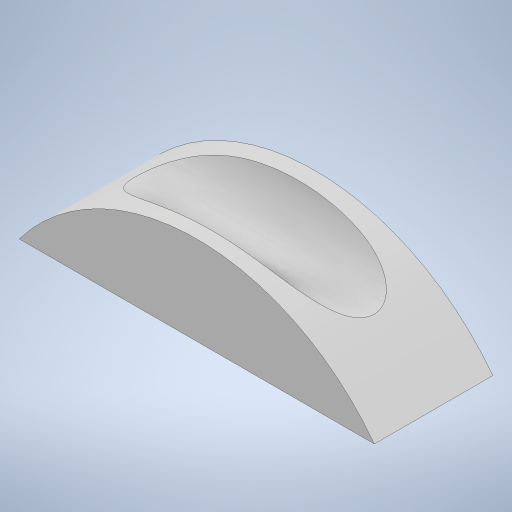
# Autodesk Inventor part: cuff
Saved by Autodesk Inventor 2024 (Build 280153000, 153)
## iProperties
Created: 2023-09-09
Part Number: cuff
Material: Generic
Document SubType Name: Modeling
Designer: Pintu
Density: 1 g/cm^3
Appearance: Default
Author: Pintu
Autodesk Inventor part; units mm, degrees
ref_plane "YZ Plane" through (0, 0, 0) normal (1, 0, 0) x (0, 1, 0)
ref_plane "XZ Plane" through (0, 0, 0) normal (0, 1, 0) x (-1, 0, 0)
ref_plane "XY Plane" through (0, 0, 0) normal (0, 0, 1) x (1, 0, 0)
sketch "Sketch1" plane through (0, 0, 0) normal (0, 0, 1) x (1, 0, 0)
  arc A0 (120, 0) -> (-120, 0) centre (0, -90) ccw
  line L0 (-120, 0) -> (120, 0)
  point P0 (0, 0)
  dimension "d0" = 240
  dimension "d1" = 150
  dimension "d2" = 120
  constraints: 2 end point, 2 horizontal alignment, 2 point on circle, 1 centre point, 1 horizontal
  measures "d0" distance of L0.start L0.end
  measures "d1" radius of A0
  measures "d2" distance of L0.start point (0, 0)
extrude "Extrusion1" add sketch "Sketch1" along normal mid plane 80
sketch "Sketch2" plane through (0, 0, 0) normal (1, 0, 0) x (0, 1, 0)
  line L0 (60, -40) -> (60, 40) projected
  arc A0 (60, 30) -> (60, -28.5626) centre (66.5274, 0.7187) ccw
  point P0 (0, 0)
  point P1 (60, 0)
  dimension "d5" = 30
  dimension "d6" = 30
  constraints: 2 point on circle, 2 point on line, 1 centre point, 1 midpoint
  measures "d5" radius of A0
  measures "d6" distance of point (60, 0) A0.start
extrude "Extrusion2" cut sketch "Sketch2" along normal mid plane 500
body "Solid1"
